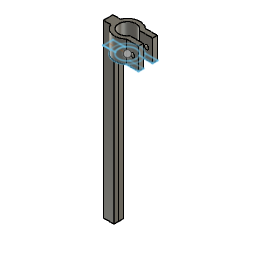
Main Hold v1 (Autodesk Fusion 360 design; units mm, degrees)
Autodesk Fusion 360 part; units mm, degrees
note: some values were not read from the file. Chosen so that the rebuilt part matches the saved one: which face or edge a step refers to. Set by a fixed rule: which sketch regions a step uses.
sketch "Sketch1" plane through (0, 0, 0) normal (0, 0, 1) x (1, 0, 0)
  line L0 (-6.8161, 4.6338) -> (-18.242, 4.6338)
  line L1 (8.001, -8.943) -> (19.5137, -8.943)
  line L2 (19.5137, -8.943) -> (19.5137, -4.443)
  line L3 (-18.242, -4.3662) -> (-6.9956, -4.3662)
  circle A0 centre (0.0069, -0.0041) radius 8.25
  arc A1 (-6.9956, -4.3662) -> (6.9609, -4.443) centre (0.0069, -0.0041) ccw
  line L4 (8.1435, 8.8053) -> (19.5137, 8.8053)
  line L5 (-11.0521, 4.6338) -> (-6.8161, 4.6338)
  line L6 (19.5137, 8.8053) -> (8.1435, 8.8053)
  line L7 (19.5137, -8.943) -> (19.5137, -4.443)
  arc A2 (-6.8161, 4.6338) -> (-6.9956, -4.3662) centre (0.0069, -0.0041) ccw
  line L8 (19.5137, 4.3053) -> (19.5137, 8.8053)
  line L9 (19.5137, 4.3053) -> (7.0419, 4.3053)
  circle A3 centre (0.0069, -0.0041) radius 12.0488
  line L10 (-18.242, 4.6338) -> (-18.242, -4.3662)
  line L11 (8.001, -8.943) -> (19.5137, -8.943)
  line L12 (19.5137, 4.3053) -> (19.5137, 8.8053)
  arc A4 (7.0419, 4.3053) -> (-6.8161, 4.6338) centre (0.0069, -0.0041) ccw
  line L13 (7.0419, 4.3053) -> (19.5137, 4.3053)
  line L14 (19.5137, -4.443) -> (6.9609, -4.443)
  line L15 (-11.0521, 4.6338) -> (-18.242, 4.6338)
  line L16 (-6.9956, -4.3662) -> (-11.1637, -4.3662)
  line L17 (-18.242, -4.3662) -> (-11.1637, -4.3662)
  line L18 (-18.242, 4.6338) -> (-18.242, -4.3662)
  line L19 (0.0069, -0.0041) -> (-18.242, -0.0041) construction
  line L20 (-8.2415, 0.1604) -> (-8.2415, -4.3662)
  line L21 (-8.2415, 0.1604) -> (-8.2415, 4.6355)
  line L22 (-8.2415, -4.3662) -> (-8.2415, 4.6355)
  dimension "d6" = 90
  constraint concentric A0 A2
  constraint concentric A0 A3
  constraint coincident L1.start L11.start
  constraint coincident L1.end L2.start
  constraint coincident L2.end L7.end
  constraint coincident L8.start L9.start
  constraint coincident L4.end L6.start
  constraint coincident L4.start L6.end
  constraint coincident L9.end A4.start
  constraint coincident L5.start L15.start
  constraint coincident L0.end L10.start
  constraint coincident L3.start L10.end
  constraint coincident L16.end L17.end
  constraint coincident A0.centre A1.centre
  constraint coincident L18 L19.end
  constraint perpendicular L18 L19
  constraint midpoint A2 L20.start
  constraint coincident L16 L20.end
  constraint coincident L3 L20.end
  constraint perpendicular L5 L21
  constraint perpendicular L0 L22
  measures "d6" angle of L19 L20
extrude "Extrude1" add sketch "Sketch1" along normal blind 20.5 contours L0 A0 L5 A2 L21 L22 | L0 A0 L5 L9 A3 A4 L13 L15 | L3 A0 A2 L16 L20 L22 | L0 L3 L5 A3 L15 L16 L17 L20 L21 L22 | L4 L6 L8 L9 A3 L12 L13 | L3 A0 A1 A3 L14 L16 L17 | L0 L3 A3 L10 L15 L17 L18 | L1 L2 L7 A3 L11 L14
sketch "Sketch2" plane through (0, 8.8053, 0) normal (0, 1, 0) x (-1, 0, 0)
  line L0 (-19.5137, 0) -> (-8.2268, 0)
  line L1 (-8.2268, 20.5) -> (-19.5137, 20.5)
  line L2 (-19.5137, 20.5) -> (-19.5137, 0)
  line L3 (-8.2268, 0) -> (-19.5137, 20.5) construction
  line L4 (-8.2268, 20.5) -> (-19.5137, 0) construction
  circle A0 centre (-13.8702, 10.25) radius 2
  line L5 (-8.2268, 0) -> (-8.2268, 20.5)
  dimension "d3" = 4
  constraint coincident L0.end L3.start
  constraint coincident L1.end L2.start
  constraint coincident L1.start L4.start
  constraint coincident L0.start L2.end
  constraint midpoint L4 A0.centre
  measures "d3" diameter of A0
extrude "Extrude2" cut sketch "Sketch2" against normal blind 39 contours A0
extrude "Extrude3" add sketch "Sketch1" against normal blind 141.5 contours L0 A0 L5 A2 L21 L22 | L3 A0 A2 L16 L20 L22 | L0 L3 L5 A3 L15 L16 L17 L20 L21 L22 | L0 L3 A3 L10 L15 L17 L18
extrude "Extrude4" cut sketch "Sketch1" against normal blind 144 contours L0 A0 L5 A2 L21 L22 | L3 A0 A2 L16 L20 L22
extrude "Extrude5" cut 2 faces at (-9.3904, -2.3691, -141.5) (-16.175, 0.1374, -141.5) along direction (0, 0, 1) blind 141
extrude "Extrude6" add 2 faces at (-9.3904, -2.3691, -0.5) (-16.175, 0.1374, -0.5) along direction (0, 0, -1) blind 141
